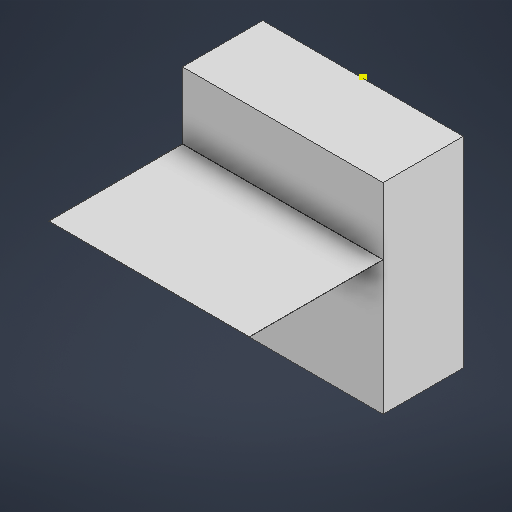
# Autodesk Inventor part: 便签
Saved by Autodesk Inventor 2025 (Build 290162000, 162)
## iProperties
Created: 2025-11-30
Part Number: 便签
Material: 常规
Document SubType Name: Modeling
Designer: XH
Density: 1 g/cm^3
Appearance: 默认
Author: XH
Autodesk Inventor part; units mm, degrees
ref_plane "YZ Plane" through (0, 0, 0) normal (1, 0, 0) x (0, 1, 0)
ref_plane "XZ Plane" through (0, 0, 0) normal (0, 1, 0) x (-1, 0, 0)
ref_plane "XY Plane" through (0, 0, 0) normal (0, 0, 1) x (1, 0, 0)
sketch "草图1" plane through (0, 0, 0) normal (0, 0, 1) x (1, 0, 0)
  line L0 (37.5, -37.5) -> (-37.5, -37.5)
  line L1 (-37.5, -37.5) -> (-37.5, 37.5)
  line L2 (-37.5, 37.5) -> (37.5, 37.5)
  line L3 (37.5, 37.5) -> (37.5, -37.5)
  line L4 (37.5, -37.5) -> (-37.5, 37.5) construction
  line L5 (-37.5, -37.5) -> (37.5, 37.5) construction
  point P0 (0, 0)
  dimension "d0" = 75
  dimension "d1" = 75
  constraints: 12 end point, 2 midpoint, 2 parallel, 1 horizontal, 1 perpendicular
  measures "d0" distance of L1.end L2.end
  measures "d1" distance of L2.end L0.start
extrude "拉伸1" add sketch "草图1" along normal blind 30
sketch "草图2" plane through (-37.5, 37.5, 0) normal (0, 1, 0) x (1, 0, 0)
  point P0 (37.5, 0)
ref_plane "工作平面1" through (-37.5, 12.5, 0) normal (0, 1, 0) x (1, 0, 0)
sketch "草图3" plane through (-37.5, 12.5, 0) normal (0, 1, 0) x (1, 0, 0)
  line L0 (75, -30) -> (0, -30) projected
  line L1 (75, -30) -> (0, -30)
  line L2 (0, -30) -> (0, -80)
  line L3 (0, -80) -> (75, -80)
  line L4 (75, -80) -> (75, -30)
  line L5 (0, 0) -> (0, -30) projected
  point P0 (37.5, 0)
  dimension "d5" = 50
  constraints: 8 end point, 2 parallel, 1 collinear, 1 horizontal, 1 perpendicular
  measures "d5" distance between parallel lines of L0 L3
extrude "拉伸2" add sketch "草图3" along normal blind 0.1
